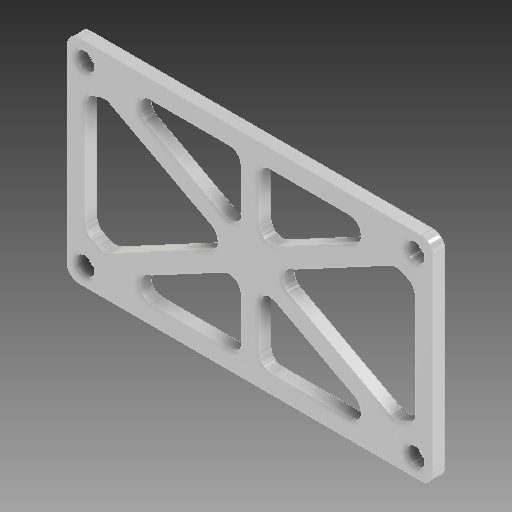
# Autodesk Inventor part: 1369-21.5-400-018 Limelight Backing
Saved by Autodesk Inventor 2022 (Build 260153000, 153)
## iProperties
Created: 2021-03-30
Part Number: 1369-21.5-400-018 Limelight Backing
Material: Aluminum 6061
Document SubType Name: Modeling
Density: 2.7 g/cm^3
Appearance: Aluminum - Dark
Autodesk Inventor part; units mm, degrees
ref_plane "YZ Plane" through (0, 0, 0) normal (1, 0, 0) x (0, 1, 0)
ref_plane "XZ Plane" through (0, 0, 0) normal (0, 1, 0) x (-1, 0, 0)
ref_plane "XY Plane" through (0, 0, 0) normal (0, 0, 1) x (1, 0, 0)
sketch "Sketch1" plane through (0, 0, 0) normal (0, 0, 1) x (1, 0, 0)
  line L0 (44.45, -23.8125) -> (-44.45, -23.8125) construction
  line L1 (-44.45, -23.8125) -> (-44.45, 23.8125) construction
  line L2 (-44.45, 23.8125) -> (44.45, 23.8125) construction
  line L3 (44.45, 23.8125) -> (44.45, -23.8125) construction
  line L4 (44.45, -23.8125) -> (-44.45, 23.8125) construction
  line L5 (-44.45, -23.8125) -> (44.45, 23.8125) construction
  circle A0 centre (-44.45, 23.8125) radius 2.4892
  circle A1 centre (44.45, 23.8125) radius 2.4892
  circle A2 centre (44.45, -23.8125) radius 2.4892
  circle A3 centre (-44.45, -23.8125) radius 2.4892
  line L6 (49.2125, -28.575) -> (-49.2125, -28.575)
  line L7 (-49.2125, -28.575) -> (-49.2125, 28.575)
  line L8 (-49.2125, 28.575) -> (49.2125, 28.575)
  line L9 (49.2125, 28.575) -> (49.2125, -28.575)
  line L10 (49.2125, -28.575) -> (-49.2125, 28.575) construction
  line L11 (-49.2125, -28.575) -> (49.2125, 28.575) construction
  point P0 (0, 0)
  dimension "d0" = 88.9
  dimension "d1" = 47.625
  dimension "d2" = 4.9784
  dimension "d3" = 98.425
  dimension "d4" = 57.15
  constraints: 24 end point, 4 centre point, 4 coincident, 4 midpoint, 4 parallel, 3 equal radius, 2 horizontal, 2 perpendicular
  measures "d0" distance of L1.end L2.end
  measures "d1" distance of L0.end L1.end
  measures "d2" diameter of A0
  measures "d3" distance of L7.end L8.end
  measures "d4" distance of L6.end L7.end
extrude "Extrusion1" add sketch "Sketch1" along normal blind 3.175
fillet "Fillet1" radius 3.175 4 edges at (-49.2125, 28.575, 1.5875) (49.2125, 28.575, 1.5875) (49.2125, -28.575, 1.5875) (-49.2125, -28.575, 1.5875)
sketch "Sketch2" plane through (0, 0, 3.175) normal (0, 0, 1) x (1, 0, 0)
  arc A0 (-49.2125, -25.4) -> (-46.0375, -28.575) centre (-46.0375, -25.4) ccw projected
  line L0 (-46.0375, -28.575) -> (46.0375, -28.575) projected
  arc A1 (46.0375, -28.575) -> (49.2125, -25.4) centre (46.0375, -25.4) ccw projected
  line L1 (49.2125, -25.4) -> (49.2125, 25.4) projected
  arc A2 (49.2125, 25.4) -> (46.0375, 28.575) centre (46.0375, 25.4) ccw projected
  line L2 (46.0375, 28.575) -> (-46.0375, 28.575) projected
  arc A3 (-46.0375, 28.575) -> (-49.2125, 25.4) centre (-46.0375, 25.4) ccw projected
  line L3 (-49.2125, 25.4) -> (-49.2125, -25.4) projected
  circle A4 centre (-44.45, -23.8125) radius 2.4892 projected
  circle A5 centre (44.45, -23.8125) radius 2.4892 projected
  circle A6 centre (44.45, 23.8125) radius 2.4892 projected
  circle A7 centre (-44.45, 23.8125) radius 2.4892 projected
  line L4 (-44.45, 23.8125) -> (44.45, 23.8125)
  line L5 (44.45, 23.8125) -> (44.45, -23.8125)
  line L6 (44.45, -23.8125) -> (-44.45, -23.8125)
  line L7 (-44.45, -23.8125) -> (-44.45, 23.8125)
  circle A8 centre (-44.45, 23.8125) radius 7.2517
  circle A9 centre (-44.45, -23.8125) radius 7.2517
  circle A10 centre (44.45, -23.8125) radius 7.2517
  circle A11 centre (44.45, 23.8125) radius 7.2517
  circle A12 centre (44.45, -23.8125) radius 2.4892 projected
  line L8 (-44.45, 23.8125) -> (44.45, -23.8125) construction
  line L9 (-45.5745, 21.7135) -> (43.3255, -25.9115)
  line L10 (45.5745, -21.7135) -> (-43.3255, 25.9115)
  arc A13 (-43.3255, 25.9115) -> (-45.5745, 21.7135) centre (-44.45, 23.8125) ccw
  arc A14 (43.3255, -25.9115) -> (45.5745, -21.7135) centre (44.45, -23.8125) ccw
  line L11 (44.45, 23.8125) -> (-44.45, -23.8125) construction
  line L12 (43.3255, 25.9115) -> (-45.5745, -21.7135)
  line L13 (-43.3255, -25.9115) -> (45.5745, 21.7135)
  arc A15 (45.5745, 21.7135) -> (43.3255, 25.9115) centre (44.45, 23.8125) ccw
  arc A16 (-45.5745, -21.7135) -> (-43.3255, -25.9115) centre (-44.45, -23.8125) ccw
  line L14 (0, 28.575) -> (0, -28.575) construction
  line L15 (-46.0375, -28.575) -> (46.0375, -28.575) projected
  line L16 (-2.3812, 28.575) -> (-2.3813, -28.575)
  line L17 (2.3813, -28.575) -> (2.3813, 28.575)
  arc A17 (2.3813, 28.575) -> (-2.3812, 28.575) centre (0, 28.575) ccw
  arc A18 (-2.3813, -28.575) -> (2.3813, -28.575) centre (0, -28.575) ccw
  point P0 (0, 0)
  point P1 (0, 0)
  point P2 (0, 0)
  point P3 (0, 0)
  point P4 (-2.3813, 3.9771)
  point P5 (-2.3812, 23.8125)
  point P6 (-37.1983, 23.8125)
  point P7 (-37.2878, 22.677)
  point P8 (2.3813, 23.8125)
  point P9 (2.3813, 3.9771)
  point P10 (37.2878, 22.677)
  point P11 (37.1983, 23.8125)
  point P12 (39.5367, 18.479)
  point P13 (5.0427, 0)
  point P14 (39.5367, -18.479)
  point P15 (44.45, -16.5608)
  point P16 (44.45, 16.5608)
  point P17 (2.3813, -3.9771)
  point P18 (2.3813, -23.8125)
  point P19 (37.1983, -23.8125)
  point P20 (37.2878, -22.677)
  point P21 (-2.3813, -23.8125)
  point P22 (-2.3813, -3.9771)
  point P23 (-37.2878, -22.677)
  point P24 (-37.1983, -23.8125)
  point P25 (-39.5367, -18.479)
  point P26 (-5.0427, 0)
  point P27 (-39.5367, 18.479)
  point P28 (-44.45, 16.5608)
  point P29 (-44.45, -16.5608)
  dimension "d8" = 4.7625
  dimension "d9" = 4.7625
  dimension "d10" = 4.7625
  dimension "d11" = 4.7625
  dimension "d12" = 4.7625
  dimension "d13" = 4.7625
  dimension "d14" = 4.7625
  dimension "d15" = 4.7625
  constraints: 32 end point, 12 point on circle, 12 tangent, 10 centre point, 5 midpoint, 3 parallel, 3 other
  measures "d8" distance between parallel lines of L2 L4
  measures "d9" radial gap between concentric circles of A7 A8
  measures "d10" radial gap between concentric circles of A4 A9
  measures "d11" radial gap between concentric circles of A5 A10
  measures "d12" radial gap between concentric circles of A6 A11
  measures "d13" diameter of A14
  measures "d14" diameter of A16
  measures "d15" diameter of A18
extrude "Extrusion2" cut sketch "Sketch2" against normal blind 3.175 contours L7 A8 L9 L12 A9 | A9 L13 L16 L6 | L4 L16 L10 A8 | L17 L9 A10 L6 | L4 A11 L12 L17 | L10 L13 A11 L5 A10
fillet "Fillet2" radius 3.175 26 edges at (37.2878, -22.677, 1.5875) (37.1983, -23.8125, 1.5875) (2.3813, -3.9771, 1.5875) (2.3813, -23.8125, 1.5875) (-37.2878, 22.677, 1.5875) (-37.1983, 23.8125, 1.5875) (-2.3813, 3.9771, 1.5875) (-2.3812, 23.8125, 1.5875) (-37.1983, -23.8125, 1.5875) (-37.2878, -22.677, 1.5875) (-2.3813, -23.8125, 1.5875) (-2.3813, -3.9771, 1.5875) (44.45, -16.5608, 1.5875) (39.5367, -18.479, 1.5875) (44.45, 16.5608, 1.5875) (39.5367, 18.479, 1.5875) (5.0427, 0, 1.5875) (37.1983, 23.8125, 1.5875) (37.2878, 22.677, 1.5875) (2.3813, 23.8125, 1.5875) (2.3813, 3.9771, 1.5875) (-44.45, 16.5608, 1.5875) (-39.5367, 18.479, 1.5875) (-44.45, -16.5608, 1.5875) (-39.5367, -18.479, 1.5875) (-5.0427, 0, 1.5875)
body "Solid1"
